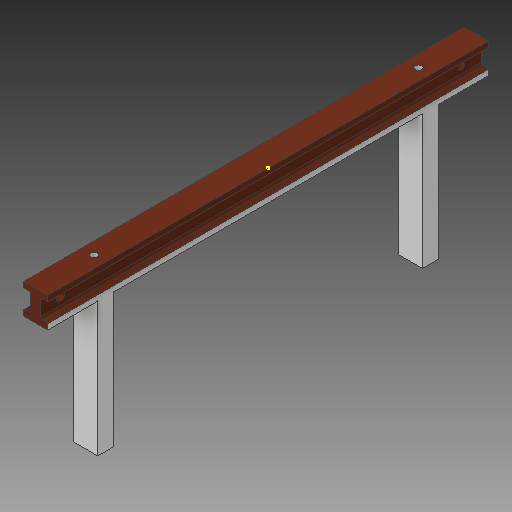
# Autodesk Inventor part: BarraEx
Saved by Autodesk Inventor 2019 (Build 230136000, 136)
## iProperties
Created: 2019-02-26
Part Number: BarraEx
Material: Generic
Document SubType Name: Modeling
Designer: felix
Density: 1 g/cm^3
Appearance: Default
Mass: 591.572 g
Surface Area: 1411.41 cm^2
Volume: 591.572 cm^3
Author: felix
Autodesk Inventor part; units mm, degrees
ref_plane "YZ Plane" through (0, 0, 0) normal (1, 0, 0) x (0, 1, 0)
ref_plane "XZ Plane" through (0, 0, 0) normal (0, 1, 0) x (-1, 0, 0)
ref_plane "XY Plane" through (0, 0, 0) normal (0, 0, 1) x (1, 0, 0)
sketch "Sketch1" plane through (0, 0, 0) normal (0, 0, 1) x (1, 0, 0)
  line L0 (0, 0) -> (-30.5, 0)
  line L1 (-30.5, 0) -> (-30.5, 38)
  line L2 (-30.5, 38) -> (0, 38)
  line L3 (0, 38) -> (0, 0)
  line L4 (0, 0) -> (0, 7)
  line L5 (0, 38) -> (0, 31)
  line L6 (0, 31) -> (-6, 31)
  line L7 (0, 7) -> (-6, 7)
  line L8 (-9, 10) -> (-9, 28)
  line L9 (-30.5, 38) -> (-30.5, 31)
  line L10 (-30.5, 31) -> (-24.5, 31)
  line L11 (-21.5, 28) -> (-21.5, 10)
  line L12 (-30.5, 0) -> (-30.5, 7)
  line L13 (-30.5, 7) -> (-24.5, 7)
  arc A0 (-6, 31) -> (-9, 28) centre (-6, 28) ccw
  arc A1 (-9, 10) -> (-6, 7) centre (-6, 10) ccw
  arc A2 (-21.5, 28) -> (-24.5, 31) centre (-24.5, 28) ccw
  arc A3 (-24.5, 7) -> (-21.5, 10) centre (-24.5, 10) ccw
  point P0 (-9, 31)
  point P1 (-21.5, 31)
  dimension "d0" = 30.5
  dimension "d1" = 38
  dimension "d2" = 7
  dimension "d3" = 7
  dimension "d4" = 9
  dimension "d6" = 7
  dimension "d7" = 9
  dimension "d8" = 7
  dimension "d9" = 3
  dimension "d11" = 3
  constraints: 28 end point, 8 point on circle, 8 point on line, 8 tangent, 4 centre point, 4 perpendicular, 3 horizontal, 3 parallel, 2 equal radius
  measures "d0" distance of L1.end L2.end
  measures "d1" distance of L0.end L1.end
  measures "d2" distance of L0.start L4.end
  measures "d3" distance of L2.end L5.end
  measures "d4" distance of L5.end point (-9, 31)
  measures "d6" distance of L1.end L9.end
  measures "d7" distance of L9.end point (-21.5, 31)
  measures "d8" distance of L0.end L12.end
  measures "d9" radius of A0
  measures "d11" radius of A2
extrude "Extrusion1" add sketch "Sketch1" along normal mid plane 558.8 contours L0 L1 L13 A3 L11 A2 L10 L2 L3 L6 A0 L8 A1 L7
hole "Hole1" at (-9, 19, 254) direction (-1, 0, 0) diameter 10 depth 25
hole "Hole2" at (-9, 19, -254) direction (-1, 0, 0) diameter 10 depth 25 tip angle 118
sketch "Sketch2" plane through (-30.5, 0, 279.4) normal (0, -1, 0) x (1, 0, 0)
  line L0 (0, 0) -> (30.5, 0) projected
  line L1 (15.25, 0) -> (15.25, -63.5)
  line L2 (15.25, -63.5) -> (0, -63.5)
  line L3 (0, -558.8) -> (0, 0) projected
  line L4 (15.25, -63.5) -> (30.5, -63.5)
  line L5 (30.5, -63.5) -> (30.5, -83.5)
  line L6 (30.5, -558.8) -> (30.5, 0) projected
  line L7 (30.5, -83.5) -> (0, -83.5)
  line L8 (0, -83.5) -> (0, -63.5)
  line L9 (30.5, -558.8) -> (0, -558.8) projected
  line L10 (15.25, -558.8) -> (15.25, -495.3)
  line L11 (15.25, -495.3) -> (30.5, -495.3)
  line L12 (15.25, -495.3) -> (0, -495.3)
  line L13 (0, -495.3) -> (0, -475.3)
  line L14 (0, -475.3) -> (30.5, -475.3)
  line L15 (30.5, -475.3) -> (30.5, -495.3)
  point P0 (30.5, -279.4)
  dimension "d33" = 63.5
  dimension "d34" = 20
  dimension "d35" = 30.5
  dimension "d36" = 63.5
  dimension "d37" = 20
  constraints: 24 end point, 8 point on line, 5 perpendicular, 2 midpoint, 2 vertical, 1 horizontal
  measures "d33" distance of L1.start L1.end
  measures "d34" distance of L4.end L5.end
  measures "d35" distance of L5.end L7.end
  measures "d36" distance of L10.start L10.end
  measures "d37" distance of L12.end L13.end
extrude "Extrusion2" add sketch "Sketch2" along normal blind 170 contours L2 L4 L5 L7 L3 | L14 L6 L11 L12 L3
sketch "Sketch5" plane through (-30.5, 38, 279.4) normal (0, 1, 0) x (1, 0, 0)
  point P0 (30.5, 279.4)
sketch "Sketch8" plane through (-30.5, -170, 279.4) normal (0, -1, 0) x (1, 0, 0)
  line L0 (30.5, -83.5) -> (30.5, -63.5) projected
  line L1 (30.5, -63.5) -> (0, -63.5) projected
  point P0 (30.5, -279.4)
  point P1 (15.5, -73.5)
  dimension "d72" = 15
  dimension "d73" = 10
  measures "d72" distance from line of L0 point (15.5, -73.5)
  measures "d73" distance from line of L1 point (15.5, -73.5)
hole "Hole5" at (-15, -170, 205.9) direction (0, 1, 0) diameter 8.647 end through all thread size "M10x1.25" class "6H" standard "ANSI Metric M Profile"
sketch "Sketch9" plane through (-30.5, -170, 279.4) normal (0, -1, 0) x (1, 0, 0)
  line L0 (30.5, -495.3) -> (30.5, -475.3) projected
  line L1 (30.5, -475.3) -> (0, -475.3) projected
  point P0 (30.5, -279.4)
  point P1 (15.5, -485.3)
  dimension "d81" = 15
  dimension "d82" = 10
  measures "d81" distance from line of L0 point (15.5, -485.3)
  measures "d82" distance from line of L1 point (15.5, -485.3)
hole "Hole6" at (-15, -170, -205.9) direction (0, 1, 0) diameter 8.647 end through all thread size "M10x1.25" class "6H" standard "ANSI Metric M Profile"
body "Solid1"
